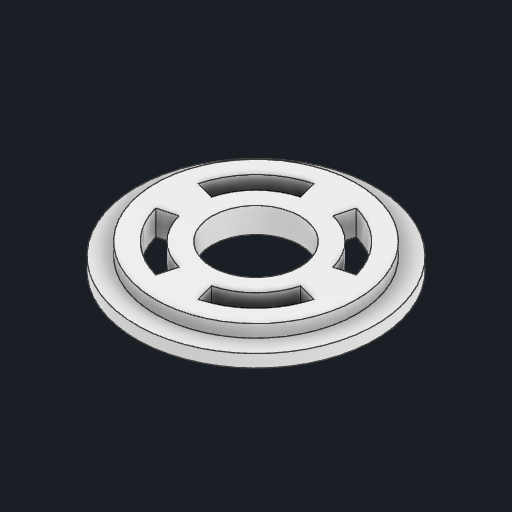
# Autodesk Inventor part: wheelcap
Saved by Autodesk Inventor 2022 (Build 260153000, 153)
## iProperties
Created: 2021-09-22
Part Number: wheelcap
Material: ABS プラスチック
Document SubType Name: Modeling
Designer: shiok
Density: 1.06 g/cm^3
Appearance: 滑らか - 白
Mass: 0.355487 g
Surface Area: 6.92112 cm^2
Volume: 0.335365 cm^3
Author: shiok
Autodesk Inventor part; units mm, degrees
ref_plane "YZ Plane" through (0, 0, 0) normal (1, 0, 0) x (0, 1, 0)
ref_plane "XZ Plane" through (0, 0, 0) normal (0, 1, 0) x (-1, 0, 0)
ref_plane "XY Plane" through (0, 0, 0) normal (0, 0, 1) x (1, 0, 0)
sketch "スケッチ1" plane through (0, 0, 0) normal (0, 1, 0) x (-1, 0, 0)
  circle A0 centre (0, 0) radius 9.5
  dimension "d0" = 19
  constraints: 1 centre point, 1 coincident
  measures "d0" diameter of A0
extrude "押し出し1" add sketch "スケッチ1" along normal blind 1
sketch "スケッチ2" plane through (0, 1, 0) normal (0, 1, 0) x (1, 0, 0)
  circle A0 centre (0, 0) radius 8
  dimension "d4" = 16
  constraints: 1 centre point, 1 coincident
  measures "d4" diameter of A0
extrude "押し出し2" add sketch "スケッチ2" along normal blind 1
sketch "スケッチ3" plane through (0, 2, 0) normal (0, 1, 0) x (1, 0, 0)
  arc A0 (-4.5962, 4.5962) -> (-6.2785, 1.6823) centre (0, 0) ccw
  line L0 (0, 0) -> (-4.5962, 4.5962) construction
  line L1 (0, 0) -> (-6.2785, 1.6823) construction
  arc A1 (-3.5355, 3.5355) -> (-4.8296, 1.2941) centre (0, 0) ccw
  line L2 (0, 0) -> (-3.5355, 3.5355) construction
  line L3 (0, 0) -> (-4.8296, 1.2941) construction
  circle A2 centre (0, 0) radius 8 projected
  line L4 (-6.2785, 1.6823) -> (-4.8296, 1.2941)
  arc A3 (-1.6823, 6.2785) -> (-4.5962, 4.5962) centre (0, 0) ccw
  arc A4 (-1.2941, 4.8296) -> (-3.5355, 3.5355) centre (0, 0) ccw
  line L5 (-1.6823, 6.2785) -> (-1.2941, 4.8296)
  line L6 (0, 0) -> (-5.3494, 0) construction
  arc A5 (-4.5962, -4.5962) -> (-1.6823, -6.2785) centre (0, 0) ccw
  line L7 (-1.6823, -6.2785) -> (-1.2941, -4.8296)
  arc A6 (-3.5355, -3.5355) -> (-1.2941, -4.8296) centre (0, 0) ccw
  arc A7 (-4.8296, -1.2941) -> (-3.5355, -3.5355) centre (0, 0) ccw
  line L8 (-6.2785, -1.6823) -> (-4.8296, -1.2941)
  arc A8 (-6.2785, -1.6823) -> (-4.5962, -4.5962) centre (0, 0) ccw
  arc A9 (4.5962, -4.5962) -> (6.2785, -1.6823) centre (0, 0) ccw
  line L9 (6.2785, -1.6823) -> (4.8296, -1.2941)
  arc A10 (3.5355, -3.5355) -> (4.8296, -1.2941) centre (0, 0) ccw
  arc A11 (1.2941, -4.8296) -> (3.5355, -3.5355) centre (0, 0) ccw
  line L10 (1.6823, -6.2785) -> (1.2941, -4.8296)
  arc A12 (1.6823, -6.2785) -> (4.5962, -4.5962) centre (0, 0) ccw
  arc A13 (4.5962, 4.5962) -> (1.6823, 6.2785) centre (0, 0) ccw
  line L11 (1.6823, 6.2785) -> (1.2941, 4.8296)
  arc A14 (3.5355, 3.5355) -> (1.2941, 4.8296) centre (0, 0) ccw
  arc A15 (4.8296, 1.2941) -> (3.5355, 3.5355) centre (0, 0) ccw
  line L12 (6.2785, 1.6823) -> (4.8296, 1.2941)
  arc A16 (6.2785, 1.6823) -> (4.5962, 4.5962) centre (0, 0) ccw
  dimension "d8" = 30
  dimension "d9" = 5
  dimension "d12" = 1.5
  dimension "d13" = 45
  dimension "d16" = 360
  constraints: 32 point on circle, 26 end point, 16 centre point, 9 coincident, 3 collinear, 2 symmetric about line, 1 horizontal, 59 other
  measures "d8" angle of L0 L1
  measures "d9" radius of A1
  measures "d12" radial gap between concentric circles of A0 A2
  measures "d13" angle of L6 L0
extrude "押し出し3" cut sketch "スケッチ3" against normal through all contours A3 L5 A4 A1 L4 A0 | A8 L8 A7 A6 L7 A5 | A12 L10 A11 A10 L9 A9 | A16 L12 A15 A14 L11 A13
sketch "スケッチ4" plane through (0, 2, 0) normal (0, 1, 0) x (1, 0, 0)
  circle A0 centre (0, 0) radius 3.5
  dimension "d20" = 7
  constraints: 1 centre point, 1 coincident
  measures "d20" diameter of A0
extrude "押し出し4" cut sketch "スケッチ4" against normal blind 10
